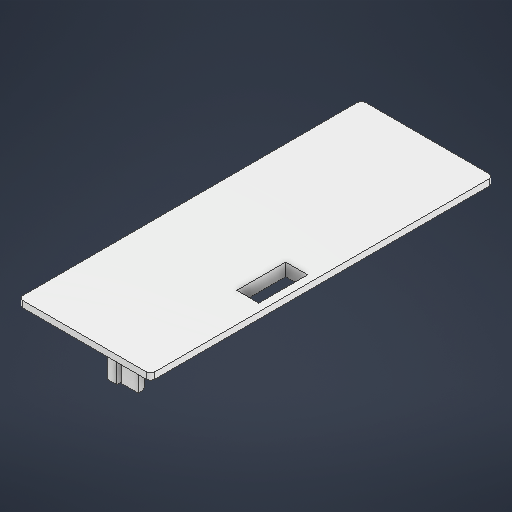
# Autodesk Inventor part: module-lid_command
Saved by Autodesk Inventor 2025.4 (Build 294407000, 407)
## iProperties
Created: 2025-09-05
Part Number: module-lid_command
Material: PC/ABS Plastic
Document SubType Name: Modeling
Designer: sam
Density: 1.1 g/cm^3
Appearance: Smooth - White
Author: sam
Autodesk Inventor part; units mm, degrees
ref_plane "YZ Plane" through (0, 0, 0) normal (1, 0, 0) x (0, 1, 0)
ref_plane "XZ Plane" through (0, 0, 0) normal (0, 1, 0) x (-1, 0, 0)
ref_plane "XY Plane" through (0, 0, 0) normal (0, 0, 1) x (1, 0, 0)
sketch "Sketch1" plane through (0, 0, 0) normal (0, 1, 0) x (-1, 0, 0)
  line L0 (-31.2, -81) -> (31.2, -81)
  line L1 (31.2, -81) -> (31.2, 81)
  line L2 (31.2, 81) -> (-31.2, 81)
  line L3 (-31.2, 81) -> (-31.2, -81)
  line L4 (-31.2, -81) -> (31.2, 81) construction
  line L5 (31.2, -81) -> (-31.2, 81) construction
  point P0 (0, 0)
  dimension "d0" = 62.4
  dimension "d1" = 162
  constraints: 12 end point, 2 midpoint, 2 parallel, 1 horizontal, 1 perpendicular
  measures "d0" distance of L2.end L1.end
  measures "d1" distance of L1.end L0.end
extrude "Extrusion1" add sketch "Sketch1" against normal blind 3
sketch "Sketch2" plane through (0, -3, 0) normal (0, -1, 0) x (1, 0, 0)
  line L0 (-31.2, 81) -> (-31.2, -81) projected
  line L1 (-31.2, -81) -> (31.2, -81) projected
  line L2 (31.2, -81) -> (31.2, 81) projected
  line L3 (31.2, 81) -> (-31.2, 81) projected
  line L4 (28, 77.8) -> (-28, 77.8)
  line L5 (-28, 77.8) -> (-28, -77.8)
  line L6 (-28, -77.8) -> (28, -77.8)
  line L7 (28, -77.8) -> (28, 77.8)
  line L8 (28, 77.8) -> (-28, -77.8) construction
  line L9 (-28, 77.8) -> (28, -77.8) construction
  point P0 (0, 0)
  dimension "d4" = 3.2
  dimension "d5" = 3.2
  constraints: 12 end point, 2 midpoint, 2 parallel, 1 horizontal, 1 perpendicular
  measures "d4" distance between parallel lines of L5 L0
  measures "d5" distance between parallel lines of L1 L6
extrude "Extrusion2" add sketch "Sketch2" along normal blind 3 contours L7 L6 L5 L4
fillet "Fillet1" radius 2 8 edges at (28, -4.5, 77.8) (-28, -4.5, 77.8) (31.2, -1.5, 81) (-31.2, -1.5, 81) (28, -4.5, -77.8) (31.2, -1.5, -81) (-28, -4.5, -77.8) (-31.2, -1.5, -81)
fillet "Fillet2" radius 0.5 8 edges at (-27.4142, -6, 77.2142) (-28, -6, 0) (-27.4142, -6, -77.2142) (0, -6, -77.8) (27.4142, -6, -77.2142) (28, -6, 0) (27.4142, -6, 77.2142) (0, -6, 77.8)
sketch "Sketch3" plane through (0, -6, 0) normal (0, -1, 0) x (1, 0, 0)
  line L0 (26, 77.8) -> (-26, 77.8) projected
  arc A0 (-26, 77.8) -> (-28, 75.8) centre (-26, 75.8) ccw projected
  arc A1 (28, 75.8) -> (26, 77.8) centre (26, 75.8) ccw projected
  line L1 (28, -75.8) -> (28, 75.8) projected
  line L2 (-28, 75.8) -> (-28, -75.8) projected
  line L3 (22.2, 77.8) -> (14.14, 77.8)
  line L4 (14.14, 77.8) -> (14.14, 74.8)
  line L5 (14.14, 74.8) -> (22.2, 74.8)
  line L6 (22.2, 74.8) -> (22.2, 77.8)
  line L7 (31.2, -79) -> (31.2, 79) projected
  point P0 (0, 0)
  point P1 (-17.6788, 77.8)
  point P2 (-8.3626, 77.8)
  dimension "d10" = 8.06
  dimension "d11" = 3
  dimension "d18" = 9
  constraints: 8 end point, 3 point on line, 2 parallel, 1 horizontal, 1 perpendicular
  measures "d10" distance of L5.end L4.end
  measures "d11" distance of L4.end L3.end
  measures "d18" distance between parallel lines of L7 L6
extrude "Extrusion3" add sketch "Sketch3" along normal blind 10.8 from surface at -3
sketch "Sketch9" plane through (0, -6, 0) normal (0, -1, 0) x (1, 0, 0)
  line L0 (14.14, 77.8) -> (-26, 77.8) projected
  line L1 (12.14, 77.8) -> (7.44, 77.8)
  line L2 (7.44, 77.8) -> (7.44, 74.8)
  line L3 (7.44, 74.8) -> (12.14, 74.8)
  line L4 (12.14, 74.8) -> (12.14, 77.8)
  line L5 (14.14, 74.8) -> (14.14, 77.8) projected
  point P0 (0, 0)
  point P1 (-1.15, 77.8)
  point P2 (11.14, 72.8)
  dimension "d57" = 4.7
  dimension "d58" = 3
  dimension "d59" = 2
  constraints: 8 end point, 2 parallel, 1 horizontal, 1 perpendicular, 1 point on line, 1 other
  measures "d57" distance of L3.end L2.end
  measures "d58" distance of L2.end L1.end
extrude "Extrusion9" add sketch "Sketch9" along normal blind 12.4 from surface at -3
sketch "Sketch7" plane through (0, 0, 0) normal (0, 1, 0) x (1, 0, 0)
  line L0 (17.2, -3.2) -> (27.6, -3.2)
  line L1 (27.6, -3.2) -> (27.6, -26.3)
  line L2 (27.6, -26.3) -> (17.2, -26.3)
  line L3 (17.2, -26.3) -> (17.2, -3.2)
  line L4 (-29.2, -81) -> (29.2, -81) projected
  line L5 (31.2, -79) -> (31.2, 79) projected
  point P0 (0, 0)
  dimension "d39" = 10.4
  dimension "d40" = 23.1
  dimension "d43" = 54.7
  dimension "d44" = 3.6
  constraints: 8 end point, 2 parallel, 1 horizontal, 1 perpendicular
  measures "d39" distance of L1.end L2.end
  measures "d40" distance of L0.end L1.end
  measures "d43" distance between parallel lines of L4 L2
  measures "d44" distance between parallel lines of L5 L1
extrude "Extrusion7" cut sketch "Sketch7" against normal through all
chamfer "Chamfer2" distance 1 angle 45 2 edges at (9.79, -15.4, 74.8) (18.17, -13.8, 74.8)
body "Solid1"
